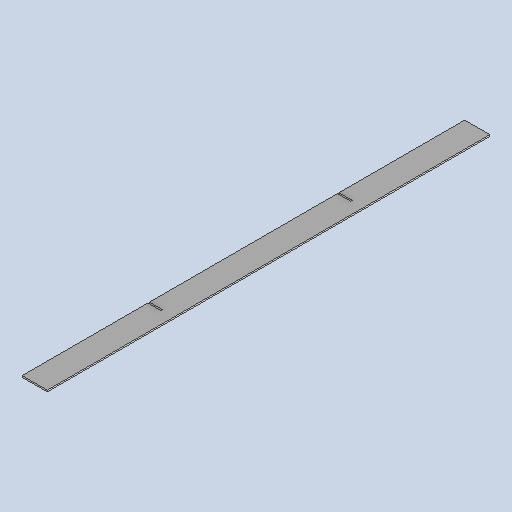
# Autodesk Inventor part: MSC 0165 rib cone exit back
Saved by Autodesk Inventor 2025 (Build 290162010, 162A)
## iProperties
Created: 2024-08-26
Part Number: MSC 0165 rib cone exit back
Material: Stainless Steel
Document SubType Name: Sheet Metal
Designer: pokla
Density: 8 g/cm^3
Sheet Metal Rule: AISI304 3mm Die 32
Appearance: Default
Stock Number: МОО 0165 шпангоут конус выход корма
Mass: 1052.26 g
Surface Area: 935.8 cm^2
Volume: 131.532 cm^3
Flat Pattern Width: 5 cm
Flat Pattern Length: 88 cm
Flat Pattern Area: 440 cm^2
Sheet Metal Width: 50,000 mm
Sheet Metal Length: 880,000 mm
Sheet Metal Area: 44000,000 mm^2
Author: pokla
Autodesk Inventor part; units mm, degrees
ref_plane "YZ Plane" through (0, 0, 0) normal (1, 0, 0) x (0, 1, 0)
ref_plane "XZ Plane" through (0, 0, 0) normal (0, 1, 0) x (-1, 0, 0)
ref_plane "XY Plane" through (0, 0, 0) normal (0, 0, 1) x (1, 0, 0)
sketch "Sketch1" plane through (0, 0, 0) normal (0, 0, 1) x (1, 0, 0)
  line L0 (-25, 0) -> (25, 0)
  line L1 (25, 0) -> (25, -880)
  line L2 (25, -880) -> (-25, -880)
  line L3 (-25, -880) -> (-25, 0)
  point P0 (0, 0)
  point P1 (0, 0)
  point P2 (-25, -1153.2713)
  dimension "d0" = 50
  dimension "d1" = 880
  measures "d0" distance of L0.start L0.end
  measures "d1" distance of L2.end L0.start
extrude "Plate1" add sketch "Sketch1" along normal mid plane 3
sketch "Sketch2" plane through (0, 0, 1.5) normal (0, 0, 1) x (1, 0, 0)
  line L0 (-25, -627) -> (1, -627)
  line L1 (1, -627) -> (1, -630)
  line L2 (1, -630) -> (-25, -630)
  line L3 (-25, -630) -> (-25, -627)
  line L4 (-25, -880) -> (-25, 0) projected
  line L5 (-25, -253) -> (1, -253)
  line L6 (1, -253) -> (1, -250)
  line L7 (1, -250) -> (-25, -250)
  line L8 (-25, -250) -> (-25, -253)
  point P0 (0, 0)
  point P1 (-25, -628.5)
  point P2 (-25, -440)
  point P3 (-25, -251.5)
  point P4 (-25, -440)
  point P5 (-25, -250)
  dimension "d15" = 188.5
  dimension "d16" = 3
  dimension "d17" = 26
  dimension "d18" = 188.5
  dimension "d19" = 26
  dimension "d20" = 3
  constraints: 16 end point, 4 midpoint, 4 parallel, 2 horizontal, 2 perpendicular, 2 point on line
  measures "d15" distance of point (-25, -440) point (-25, -628.5)
  measures "d16" distance of L2.end L0.start
  measures "d17" distance of L1.end L2.end
  measures "d18" distance of point (-25, -251.5) point (-25, -440)
  measures "d19" distance of L5.start L5.end
  measures "d20" distance of L5.end L6.end
extrude "Extrusion1" cut sketch "Sketch2" against normal through all
equation "\"d18\" = d15"
equation "\"d20\" = d16"
equation "\"d2\" = Thickness"
equation "\"BendReliefWidth\" = Thickness"
equation "\"BendReliefDepth\" = 0.5 * Thickness"
equation "\"CornerReliefSize\" = 4 * Thickness"
equation "\"MinimumRemnant\" = 2 * Thickness"
equation "\"TransitionRadius\" = BendRadius"
equation "\"JacobiRadiusSize\" = BendRadius"
equation "\"GapSize\" = Thickness"
equation "\"Thickness\" = 3"
equation "\"BendRadius\" = 5"
body "Solid1"
